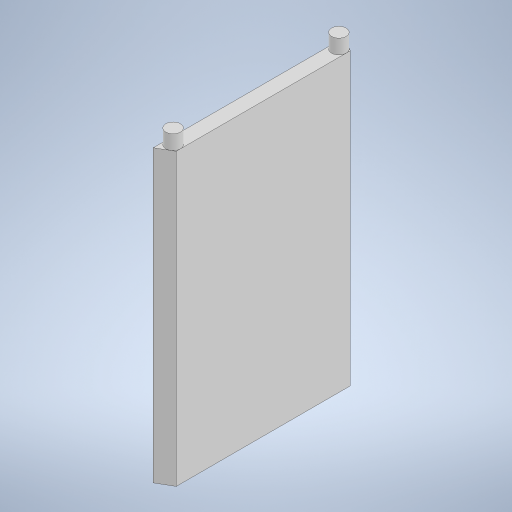
# Autodesk Inventor part: col
Saved by Autodesk Inventor 2024 (Build 280153000, 153)
## iProperties
Created: 2024-03-18
Part Number: col
Material: 일반
Document SubType Name: Modeling
Designer: SSAFY
Density: 1 g/cm^3
Appearance: 기본값
Author: SSAFY
Autodesk Inventor part; units mm, degrees
ref_plane "YZ Plane" through (0, 0, 0) normal (1, 0, 0) x (0, 1, 0)
ref_plane "XZ Plane" through (0, 0, 0) normal (0, 1, 0) x (-1, 0, 0)
ref_plane "XY Plane" through (0, 0, 0) normal (0, 0, 1) x (1, 0, 0)
sketch "스케치2" plane through (0, 0, 0) normal (0, 1, 0) x (-1, 0, 0)
  line L0 (0, -60) -> (-51.9615, -30)
  line L1 (-51.9615, -30) -> (-51.9615, 30)
  line L2 (-51.9615, 30) -> (0, 60)
  line L3 (0, 60) -> (51.9615, 30)
  line L4 (51.9615, 30) -> (51.9615, -30)
  line L5 (51.9615, -30) -> (0, -60)
  line L6 (0, -65.7735) -> (-56.9615, -32.8868)
  line L7 (-56.9615, -32.8868) -> (-56.9615, 32.8868)
  line L8 (-56.9615, 32.8868) -> (0, 65.7735)
  line L9 (0, 65.7735) -> (56.9615, 32.8868)
  line L10 (56.9615, 32.8868) -> (56.9615, -32.8868)
  line L11 (56.9615, -32.8868) -> (0, -65.7735)
  line L12 (51.9615, -30) -> (56.9615, -32.8868)
  line L13 (56.9615, 32.8868) -> (51.9615, 30)
  point P0 (0, 0)
  point P1 (0, 0)
  dimension "d0" = 60
  dimension "d1" = 5
  constraints: 28 end point, 1 coincident, 18 other
  measures "d0" distance of L3.end L4.end
  measures "d1" distance between parallel lines of L4 L10
extrude "돌출1" add sketch "스케치2" along normal blind 100 contours L4 L13 L10 L12
sketch "스케치3" plane through (0, 100, 0) normal (0, 1, 0) x (1, 0, 0)
  line L0 (-56.9615, -32.8868) -> (-51.9615, -30) construction
  line L1 (-51.9615, 30) -> (-56.9615, 32.8868) construction
  line L2 (-56.9615, 32.8868) -> (-56.9615, -32.8868) construction
  circle A0 centre (-54.4615, 28.5566) radius 2.5
  circle A1 centre (-54.4615, -28.5566) radius 2.5
  point P0 (0, 0)
  dimension "d4" = 5
  dimension "d5" = 5
  constraints: 4 tangent, 2 centre point
  measures "d4" diameter of A0
  measures "d5" diameter of A1
extrude "돌출2" add sketch "스케치3" along normal blind 5
